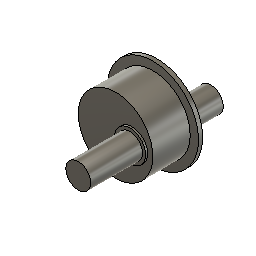
エキセントリックシャフト v15 (Autodesk Fusion 360 design; units mm, degrees)
Autodesk Fusion 360 part; units mm, degrees
sketch "スケッチ1" plane through (0, 0, 0) normal (0, 0, 1) x (1, 0, 0)
  circle A0 centre (0, 0) radius 3
  line L0 (0, 0) -> (-4, 0)
  circle A1 centre (-4, 0) radius 9
  circle A2 centre (0, 0) radius 4
  dimension "d1" = 6
  dimension "d2" = 4
  dimension "d3" = 18
  dimension "d14" = 8
  constraint coincident A0.centre L0.start
  constraint horizontal L0
  constraint coincident L0.end A1.centre
  constraint concentric A0 A2
  measures "d1" diameter of A0
  measures "d2" distance of A0.centre L0.end
  measures "d3" diameter of A1
  measures "d14" diameter of A2
extrude "押し出し1" add sketch "スケッチ1" against normal blind 10 contours A0
extrude "押し出し2" add sketch "スケッチ1" along normal blind 17 contours A0 | A1 | A2
sketch "スケッチ2" plane through (0, 0, 17) normal (0, 0, 1) x (1, 0, 0)
  circle A0 centre (-4, 0) radius 9
  circle A1 centre (0, 0) radius 3
  circle A2 centre (0, 0) radius 4
  dimension "d8" = 6
  dimension "d11" = 8
  constraint coincident A1.centre A2.centre
  measures "d8" diameter of A1
  measures "d11" diameter of A2
extrude "押し出し3" add sketch "スケッチ2" along normal blind 10 contours A1
extrude "押し出し4" add sketch "スケッチ2" along normal blind 1.5 contours A2
extrude "押し出し5" add sketch "スケッチ1" against normal blind 1.5 contours A2
extrude "押し出し6" cut sketch "スケッチ2" against normal blind 5 contours A0
extrude "押し出し7" cut 1 faces at (3.6406, -0.3478, 18.5) along direction (0, 0, -1) blind 5
extrude "押し出し8" cut 1 faces at (-9.9665, 0.4471, 12) along direction (0, 0, -1) blind 3.5
extrude "押し出し9" cut 1 faces at (3.6406, -0.3478, 13.5) along direction (0, 0, -1) blind 3.5
extrude "押し出し10" cut 1 faces at (0.3505, -0.866, 27) along direction (0, 0, -1) blind 5
extrude "押し出し11" add 1 faces at (3.6406, -0.3478, 10) along direction (0, 0, 1) blind 5
extrude "押し出し12" cut 1 faces at (-9.9665, 0.4471, 8.5) along direction (0, 0, -1) blind 1.5
extrude "押し出し13" add 1 faces at (-9.9665, 0.4471, 7) along direction (0, 0, 1) blind 1
extrude "押し出し14" cut 1 faces at (3.6406, -0.3478, 15) along direction (0, 0, -1) blind 6.5
extrude "押し出し15" add 1 faces at (3.6406, -0.3478, 8.5) along direction (0, 0, 1) blind 0.5
extrude "押し出し16" cut 1 faces at (3.6406, -0.3478, 9) along direction (0, 0, -1) blind 0.5
extrude "押し出し17" add 1 faces at (3.6406, -0.3478, 8.5) along direction (0, 0, 1) blind 0.5
sketch "スケッチ3" plane through (0, 0, 0) normal (0, 0, 1) x (1, 0, 0)
  circle A0 centre (-4, 0) radius 11
  circle A1 centre (-4, 0) radius 9
  dimension "d41" = 22
  constraint concentric A0 A1
  measures "d41" diameter of A0
extrude "押し出し18" add sketch "スケッチ3" against normal blind 1 contours A0 | A1
extrude "押し出し19" add 1 faces at (3.6406, -0.3478, 9) along direction (0, 0, 1) blind 2
extrude "押し出し20" add 1 faces at (-9.9665, 0.4471, 8) along direction (0, 0, 1) blind 2
extrude "押し出し21" cut 1 faces at (3.6406, -0.3478, 11) along direction (0, 0, -1) blind 1
extrude "押し出し22" cut 1 faces at (-9.6332, 0.4471, 10) along direction (0, 0, -1) blind 1
sketch "スケッチ4" plane through (0, 0, 9) normal (0, 0, 1) x (1, 0, 0)
  circle A0 centre (0, 0) radius 3
  circle A1 centre (-4, 0) radius 9
  circle A2 centre (0, 0) radius 3.75
  dimension "d52" = 7.5
  constraint concentric A0 A2
  measures "d52" diameter of A2
extrude "押し出し23" add sketch "スケッチ4" along normal blind 0.5 contours A2
